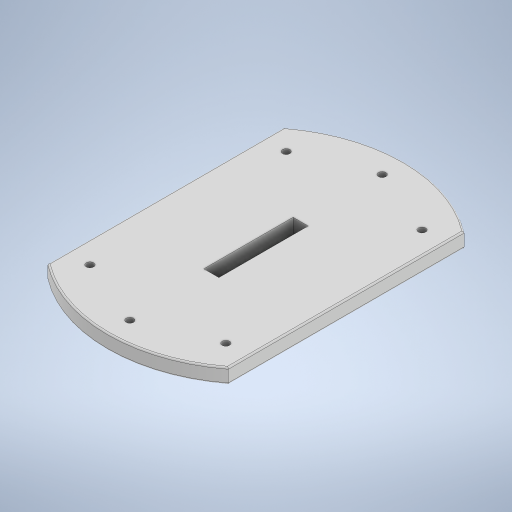
# Autodesk Inventor part: Chasis_Cap
Saved by Autodesk Inventor 2024 (Build 280153000, 153)
## iProperties
Created: 2024-06-21
Part Number: Chasis_Cap
Material: Generic
Document SubType Name: Modeling
Designer: sml6042
Density: 1 g/cm^3
Appearance: Default
Author: sml6042
Autodesk Inventor part; units mm, degrees
ref_plane "YZ Plane" through (0, 0, 0) normal (1, 0, 0) x (0, 1, 0)
ref_plane "XZ Plane" through (0, 0, 0) normal (0, 1, 0) x (-1, 0, 0)
ref_plane "XY Plane" through (0, 0, 0) normal (0, 0, 1) x (1, 0, 0)
sketch "Sketch1" plane through (0, 0, 0) normal (0, 1, 0) x (-1, 0, 0)
  circle A0 centre (0, 0) radius 50
  line L0 (-25.38, 0) -> (-25.38, 35.55)
  line L1 (-25.38, 35.55) -> (0, 35.55)
  line L2 (25.38, 35.55) -> (0, 35.55)
  line L3 (25.38, 35.55) -> (25.38, 0)
  line L4 (-25.38, 0) -> (-25.38, -35.55)
  line L5 (-25.38, -35.55) -> (0, -35.55)
  line L6 (25.38, -35.55) -> (0, -35.55)
  line L7 (25.38, -35.55) -> (25.38, 0)
  line L8 (-25.38, -35.55) -> (-25.38, -33.05)
  line L9 (-25.38, -33.05) -> (-22.88, -33.05)
  circle A1 centre (-22.88, -33.05) radius 1.25
  line L10 (-25.38, 35.55) -> (-25.38, 33.05)
  line L11 (-25.38, 33.05) -> (-22.88, 33.05)
  circle A2 centre (-22.88, 33.05) radius 1.25
  line L12 (25.38, 35.55) -> (25.38, 33.05)
  line L13 (25.38, 33.05) -> (22.88, 33.05)
  circle A3 centre (22.88, 33.05) radius 1.25
  line L14 (25.38, -35.55) -> (25.38, -33.05)
  line L15 (25.38, -33.05) -> (22.88, -33.05)
  circle A4 centre (22.88, -33.05) radius 1.25
  dimension "d0" = 100
  dimension "d4" = 50.76
  dimension "d5" = 2.5
  dimension "d6" = 2.5
  dimension "d7" = 2.5
  dimension "d8" = 2.5
  dimension "d9" = 2.5
  dimension "d10" = 2.5
  dimension "d11" = 2.5
  dimension "d12" = 2.5
  dimension "d13" = 2.5
  dimension "d14" = 2.5
  dimension "d15" = 2.5
  dimension "d16" = 2.5
  constraints: 32 end point, 8 perpendicular, 8 point on line, 5 centre point, 5 coincident, 2 collinear
  measures "d0" diameter of A0
  measures "d4" distance of L3.end L0.start
  measures "d5" distance of L4.end L8.end
  measures "d6" distance of L8.end L9.end
  measures "d7" diameter of A1
  measures "d8" distance of L0.end L10.end
  measures "d9" distance of L10.end L11.end
  measures "d10" diameter of A2
  measures "d11" distance of L2.start L12.end
  measures "d12" distance of L12.end L13.end
  measures "d13" diameter of A3
  measures "d14" distance of L6.start L14.end
  measures "d15" distance of L14.end L15.end
  measures "d16" diameter of A4
extrude "Extrusion1" add sketch "Sketch1" along normal blind 5 contours A0 | L0 L1 L2 L3 L7 L6 L5 L4
sketch "Sketch2" plane through (0, 5, 0) normal (0, 1, 0) x (1, 0, 0)
  line L0 (0, 0) -> (-2.55, 0)
  line L1 (-2.55, 0) -> (2.55, 0)
  line L2 (2.55, 0) -> (2.55, -15.05)
  line L3 (2.55, -15.05) -> (2.55, 15.05)
  line L4 (2.55, 15.05) -> (-2.55, 15.05)
  line L5 (-2.55, 15.05) -> (-2.55, -15.05)
  line L6 (-2.55, -15.05) -> (2.55, -15.05)
  dimension "d19" = 2.55
  dimension "d20" = 5.1
  dimension "d21" = 15.05
  dimension "d22" = 30.1
  constraints: 14 end point, 4 perpendicular, 2 point on line, 1 horizontal
  measures "d19" distance of L0.start L0.end
  measures "d20" distance of L0.end L1.end
  measures "d21" distance of L1.end L2.end
  measures "d22" distance of L2.end L3.end
extrude "Extrusion2" cut sketch "Sketch2" against normal blind 5
sketch "Sketch3" plane through (0, 5, 0) normal (0, 1, 0) x (1, 0, 0)
  circle A0 centre (-22.88, -33.05) radius 1.25 projected
  line L0 (-22.88, -33.05) -> (-30.38, -33.05)
  line L1 (-30.38, -33.05) -> (-30.38, -39.7122)
  circle A1 centre (0, 0) radius 50 projected
  line L2 (-30.38, -33.05) -> (-30.38, 39.7122)
  circle A2 centre (22.88, 33.05) radius 1.25 projected
  line L3 (22.88, 33.05) -> (30.38, 33.05)
  line L4 (30.38, 33.05) -> (30.38, 39.7122)
  line L5 (30.38, 39.7122) -> (30.38, -39.7122)
  dimension "d25" = 7.5
  dimension "d26" = 7.5
  constraints: 12 end point, 2 horizontal, 2 perpendicular, 2 point on circle, 2 point on line
  measures "d25" distance of L0.start L0.end
  measures "d26" distance of L3.start L3.end
extrude "Extrusion3" cut sketch "Sketch3" against normal blind 5 contours L1 A1 L2 | L5 L4 A1
sketch "Sketch4" plane through (0, 5, 0) normal (0, 1, 0) x (1, 0, 0)
  arc A0 (-30.38, -39.7122) -> (30.38, -39.7122) centre (0, 0) ccw projected
  line L0 (0, -50) -> (0, -42.5)
  circle A1 centre (0, -42.5) radius 1.25
  arc A2 (30.38, 39.7122) -> (-30.38, 39.7122) centre (0, 0) ccw projected
  line L1 (0, 50) -> (0, 42.5)
  circle A3 centre (0, 42.5) radius 1.25
  dimension "d29" = 7.5
  dimension "d30" = 2.5
  dimension "d31" = 7.5
  dimension "d32" = 2.5
  constraints: 4 end point, 2 centre point, 2 coincident, 2 point on circle, 2 vertical
  measures "d29" distance of L0.start L0.end
  measures "d30" diameter of A1
  measures "d31" distance of L1.start L1.end
  measures "d32" diameter of A3
extrude "Extrusion4" cut sketch "Sketch4" against normal blind 5
fillet "Fillet1" radius 0.5 4 edges at (0, 5, 50) (0, 5, -50) (0, 0, 50) (0, 0, -50)
body "Solid1"
